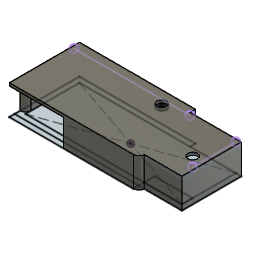
CNC_limit_switch_case_body (Autodesk Fusion 360 design; units mm, degrees)
Autodesk Fusion 360 part; units mm, degrees
note: some values were not read from the file. Chosen so that the rebuilt part matches the saved one: which face or edge a step refers to; which pieces of a blend or face edit are solid. Set by a fixed rule: which sketch regions a step uses.
sketch "Sketch1" plane through (0, 0, 0) normal (0, 1, 0) x (1, 0, 0)
  line L0 (29, 10) -> (-29, 10)
  line L1 (-29, -10) -> (29, -10)
  line L2 (29, -10) -> (29, 10)
  line L3 (29, 10) -> (-29, -10) construction
  line L4 (-29, 10) -> (29, -10) construction
  line L5 (12, 12) -> (-31, 12)
  line L6 (-31, -12) -> (31, -12)
  line L7 (31, -12) -> (31, 10)
  line L8 (29, 10) -> (31, 10)
  line L9 (12, 12) -> (12, 10)
  line L10 (-29, 10) -> (-29, -10)
  line L11 (-31, -12) -> (-31, 12)
  line L12 (29, -10) -> (15, -10)
  line L13 (15, -10) -> (15, -6.1)
  line L14 (15, -6.1) -> (29, -6.1)
  line L15 (29, -6.1) -> (29, -10)
  line L16 (15, -10) -> (15, -12)
  line L17 (15, -12) -> (15, -14)
  line L18 (15, -14) -> (-30.9998, -14)
  line L19 (-30.9998, -14) -> (-31, -14)
  line L20 (-31, -14) -> (-31, -12)
  dimension "d1" = 58
  dimension "d2" = 20
  dimension "d3" = 2
  dimension "d5" = 2
  dimension "d6" = 2
  dimension "d7" = 17
  dimension "d8" = 58
  dimension "d9" = 43
  dimension "d10" = 62
  dimension "d29" = 14
  dimension "d30" = 16.1
  dimension "d31" = 45.9998
  dimension "d32" = 2
  constraint horizontal L0
  constraint parallel L0 L1
  constraint coincident L3 origin
  constraint coincident L4 origin
  constraint perpendicular L5 L7
  constraint parallel L1 L6
  constraint perpendicular L7 L8
  constraint coincident L0 L9.end
  constraint perpendicular L0 L9
  constraint horizontal L12
  constraint vertical L13
  constraint horizontal L14
  constraint vertical L15
  constraint coincident L6 L16.end
  constraint perpendicular L6 L16
  constraint perpendicular L6 L17
  constraint perpendicular L11 L18
  constraint parallel L17 L20
  measures "d1" distance of L1.start L1.end
  measures "d2" distance of L0.end L1.start
  measures "d3" distance of L0 L5
  measures "d5" distance of L1 L6
  measures "d6" distance of L2 L7
  measures "d7" distance of L2 L9
  measures "d8" distance of L0.start L0.end
  measures "d9" distance of L5.start L5.end
  measures "d10" distance of L6.start L6.end
  measures "d29" distance of L1.end L12.end
  measures "d30" distance of L0 L14
  measures "d31" distance of L17.end L18.end
  measures "d32" distance of L6 L18
extrude "Extrude1" add sketch "Sketch1" along normal blind 10 contours L1 L2 L6 L7 L8 L12 L15 L16 | L0 L1 L5 L6 L9 L10 L11 L16 | L1 L2 L12 L13 L14 L15 | L6 L17 L18 L20 makes body 1
extrude "Extrude2" add sketch "Sketch1" along normal blind 1 from surface at 10 separate body contours L0 L1 L2 L10 L13 L14 | L1 L2 L6 L7 L8 L12 L15 L16 | L0 L1 L5 L6 L9 L10 L11 L16 | L1 L2 L12 L13 L14 L15 makes body 2
sketch "Sketch2" plane through (-31, 0, 0) normal (-1, 0, 0) x (0, 0, 1)
  line L0 (-12, 0) -> (14, 0)
  line L1 (14, 10) -> (-12, 10)
  line L2 (-12, 10) -> (-12, 0)
  line L3 (-10, 0) -> (10, 0)
  line L4 (10, 0) -> (10, 10)
  line L5 (10, 10) -> (-10, 10)
  line L6 (-10, 10) -> (-10, 0)
  line L7 (14, 0) -> (14, 10)
  dimension "d16" = 20
  constraint horizontal L3
  constraint vertical L4
  constraint horizontal L5
  constraint vertical L6
  constraint coincident L1 L4.end
  constraint coincident L0 L3.start
  measures "d16" distance of L4 L6
extrude "Extrude3" cut sketch "Sketch2" against normal blind 2 contours L0 L1 L3 L4 L5 L6 bodies 1 makes body 3 at (-15.3333, 6.6667, -10)
hole "Hole1" at (26.5, 11, 3.5) direction (0, -1, 0) diameter 3.5 depth 20 tip angle 180 bodies 2
sketch "Sketch3" plane through (0, 10, 0) normal (0, -1, 0) x (1, 0, 0)
  circle A0 centre (26.5, 3.5) radius 1.75
  line L0 (31, -10) -> (31, 12)
  line L1 (31, 12) -> (-31, 12)
  line L2 (-31, 12) -> (-31, -12)
  line L3 (-31, -12) -> (12, -12)
  line L4 (12, -12) -> (12, -10)
  line L5 (12, -10) -> (31, -10)
  circle A1 centre (4, -7.5) radius 1.75
  line L6 (29, 6.1) -> (29, -10)
  line L7 (-31, -10) -> (12, -10)
  dimension "d24" = 25
  dimension "d25" = 2.5
  dimension "d26" = 3.5
  measures "d24" distance of A1.centre L6
  measures "d25" distance of A1.centre L7
  measures "d26" diameter of A1
extrude "Extrude4" cut sketch "Sketch3" against normal blind 2 contours A1 bodies 2
extrude "Extrude5" add 1 faces at (25, 10, 10.0333) along direction (0, 1, 0) blind 1 on bodies 1 bodies 1 3 2
sketch "Sketch4" plane through (-31, 0, 0) normal (-1, 0, 0) x (0, 0, 1)
  line L0 (10, 10) -> (10, 0)
  line L1 (10, 0) -> (14, 0)
  line L2 (14, 0) -> (14, 11)
  line L3 (14, 11) -> (-12, 11)
  line L4 (-12, 11) -> (-12, 10)
  line L5 (-12, 10) -> (10, 10)
  line L6 (10, 0) -> (12, 0)
  line L7 (12, 0) -> (12, 10)
  line L8 (12, 10) -> (10, 10)
  line L9 (10, 10) -> (10, 0)
  constraint horizontal L6
  constraint vertical L7
  constraint horizontal L8
  constraint vertical L9
  constraint coincident L0.end L1.start
extrude "Extrude6" cut sketch "Sketch4" against normal blind 46 contours L0 L1 L6 L7 L8 L9 bodies 1
extrude "Extrude7" add 1 faces at (15, 7, 13.3333) along direction (1, 0, 0) blind 2 on bodies 1 bodies 1
fillet "Fillet1" radius 2 3 edges at (17, 11, 13) (17, 5.5, 14) (17, 0, 13) on bodies 1
sketch "Sketch5" plane through (-31, 0, 0) normal (-1, 0, 0) x (0, 0, 1)
  line L0 (-12, 10) -> (12, 10)
  line L1 (12, 10) -> (12, 0)
  line L2 (12, 0) -> (14, 0)
  line L3 (14, 0) -> (14, 11)
  line L4 (14, 11) -> (-12, 11)
  line L5 (-12, 11) -> (-12, 10)
  line L6 (12, 0) -> (14, 0)
  line L7 (14, 0) -> (14, 10)
  line L8 (14, 10) -> (12, 10)
  line L9 (12, 10) -> (12, 0)
  dimension "d41" = 10
  constraint horizontal L6
  constraint vertical L7
  constraint horizontal L8
  constraint vertical L9
  constraint coincident L3 L7.end
  constraint coincident L1.end L2.start
  measures "d41" distance of L6 L8
extrude "Extrude8" cut sketch "Sketch5" against normal blind 20 contours L1 L2 L3 L6 L7 L8 L9 bodies 1
sketch "Sketch6" plane through (0, 0, -10) normal (0, 0, 1) x (1, 0, 0)
  line L0 (-31, 0) -> (12, 0)
  line L1 (12, 0) -> (12, 10)
  line L2 (12, 10) -> (-31, 10)
  line L3 (-31, 10) -> (-31, 0)
  line L4 (-31, 0) -> (-29, 0)
  line L5 (-29, 0) -> (-29, 10)
  line L6 (-29, 10) -> (-31, 10)
  line L7 (-31, 10) -> (-31, 0)
  dimension "d44" = 2
  dimension "d45" = 10
  constraint horizontal L4
  constraint vertical L5
  constraint horizontal L6
  constraint vertical L7
  constraint coincident L0.start L3.end
  measures "d44" distance of L0.start L4.end
  measures "d45" distance of L0.start L2.end
extrude "Extrude9" add sketch "Sketch6" along normal blind 20 contours L0 L2 L3 L4 L5 L6 L7 bodies 1 3
fillet "Fillet2" radius 2 1 edges at (-11, 5, 12) on bodies 1
fillet "Fillet3" radius 2 1 edges at (-29, 5, 10) on bodies 1
fillet "Fillet4" radius 5 1 edges at (-29, 5, -10) on bodies 1
fillet "Fillet5" radius 2 1 edges at (15, 5, 6.1) on bodies 1
extrude "Extrude10" add sketch "Sketch1" against normal blind 1 separate body makes body 4
extrude "Extrude11" cut sketch "Sketch3" along normal blind 23 contours A1 bodies 4
extrude "Extrude12" cut sketch "Sketch3" along normal blind 20 contours A0 bodies 4
hidden bodies 4
